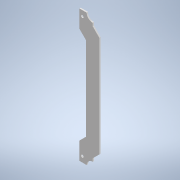
# Autodesk Inventor part: domePlace
Saved by Autodesk Inventor 2022 (Build 260153000, 153)
## iProperties
Created: 2021-07-01
Part Number: domePlace
Material: Generic
Document SubType Name: Modeling
Designer: dsdan
Density: 1 g/cm^3
Appearance: Default
Author: dsdan
Autodesk Inventor part; units mm, degrees
ref_plane "YZ Plane" through (0, 0, 0) normal (1, 0, 0) x (0, 1, 0)
ref_plane "XZ Plane" through (0, 0, 0) normal (0, 1, 0) x (-1, 0, 0)
ref_plane "XY Plane" through (0, 0, 0) normal (0, 0, 1) x (1, 0, 0)
sketch "Sketch1" plane through (0, 0, 0) normal (0, 0, 1) x (1, 0, 0)
  circle A0 centre (0, 0) radius 12.5
  circle A1 centre (0, -298.822) radius 12.5
  line L0 (-114.8008, 0.589) -> (0, 0.589)
  line L1 (0, 0.589) -> (0, -19.411)
  line L2 (0, -299.411) -> (-114.8008, -299.411)
  line L3 (-114.8008, -299.411) -> (-114.8008, 0.589) construction
  line L4 (-114.8008, 0.589) -> (0, -299.411) construction
  line L5 (0, 0.589) -> (-114.8008, -299.411) construction
  line L6 (-114.8008, -2.4111) -> (-114.8008, -296.4111) construction
  line L7 (0, -19.411) -> (15, -34.411)
  line L8 (15, -34.411) -> (15, -264.411)
  line L9 (15, -264.411) -> (0, -279.411)
  line L10 (-30, 0.589) -> (-30, -39.411)
  line L11 (-30, -39.411) -> (-15, -54.411)
  line L12 (-15, -54.411) -> (-15, -244.411)
  line L13 (-15, -244.411) -> (-30, -259.411)
  line L14 (-30, -259.411) -> (-30, -299.411)
  circle A2 centre (-22.6008, -11.9111) radius 3
  circle A3 centre (-22.6008, -286.9111) radius 3
  circle A4 centre (-22.6008, -286.9111) radius 3.5 construction
  circle A5 centre (-22.6008, -11.9111) radius 3.5 construction
  line L15 (0, -279.411) -> (0, -299.411)
  point P0 (-57.4004, -149.411)
  point P1 (12.4861, 0.589)
  point P2 (-12.4861, 0.589)
  point P3 (-12.4861, -299.411)
  point P4 (12.4861, -299.411)
  point P5 (2, -286.483)
  point P6 (0, -12.5)
  point P7 (0, -286.322)
  dimension "d0" = 25
  dimension "d1" = 25
  dimension "d2" = 298.822
  dimension "d3" = 300
  dimension "d4" = 149.411
  dimension "d6" = 149.411
  dimension "d12" = 20
  dimension "d13" = 20
  dimension "d14" = 15
  dimension "d15" = 45
  dimension "d16" = 45
  dimension "d17" = 40
  dimension "d18" = 40
  dimension "d19" = 30
  dimension "d21" = 6
  dimension "d22" = 6
  dimension "d23" = 0
  dimension "d24" = 15
  dimension "d25" = 45
  dimension "d26" = 45
  constraints: 30 end point, 5 point on line, 4 centre point, 3 coincident, 3 parallel, 3 vertical, 2 midpoint, 2 perpendicular, 1 collinear, 1 horizontal, 1 vertical alignment
  measures "d0" diameter of A0
  measures "d1" diameter of A1
  measures "d2" distance of A1.centre A0.centre
  measures "d3" distance between parallel lines of L0 L2
  measures "d4" vertical distance of A0.centre point (-57.4, -149.411)
  measures "d6" vertical distance of A1.centre point (-57.4, -149.411)
  measures "d12" distance from line of L0 L1.end
  measures "d13" distance from line of L2 L9.end
  measures "d14" distance between parallel lines of L1 L8
  measures "d15" angle of L10 L11
  measures "d16" angle of L14 L13
  measures "d17" distance of L10.start L10.end
  measures "d18" distance of L13.end L14.end
  measures "d19" distance between parallel lines of L1 L10
  measures "d21" diameter of A2
  measures "d22" diameter of A3
  measures "d23" distance from line of point (0, 0) L1
  measures "d24" distance between parallel lines of L10 L12
  measures "d25" angle of L15 L9
  measures "d26" angle of L1 L7
extrude "Extrusion1" add sketch "Sketch1" along normal blind 3 contours A0 L1 L7 L8 L9 L15 A1 L2 L14 L13 L12 L11 L10 L0
equation "\"d4\" = d6"
equation "\"d18\" = d17"
body "Solid1"
